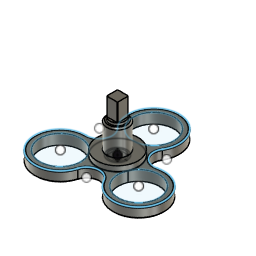
Base3 v0 (Autodesk Fusion 360 design; units mm, degrees)
Autodesk Fusion 360 part; units mm, degrees
sketch "Sketch1" plane through (0, 0, 0) normal (0, 0, 1) x (1, 0, 0)
  circle A0 centre (0, 0) radius 4
  circle A1 centre (0, 0) radius 1.5
  line L0 (0.98, 1.06) -> (-0.98, 1.06)
  line L1 (-1.06, 0.98) -> (-1.06, -0.98)
  line L2 (-0.98, -1.06) -> (0.98, -1.06)
  line L3 (1.06, -0.98) -> (1.06, 0.98)
  line L4 (1.06, 1.06) -> (-1.06, -1.06) construction
  line L5 (-1.06, 1.06) -> (1.06, -1.06) construction
  line L6 (0.98, 1.06) -> (1.06, 0.98)
  line L7 (-0.98, 1.06) -> (-1.06, 0.98)
  line L8 (-1.06, -0.98) -> (-0.98, -1.06)
  line L9 (1.06, -0.98) -> (0.98, -1.06)
  circle A2 centre (-0.8867, 7.9507) radius 4
  circle A3 centre (-6.4421, -4.7433) radius 4
  circle A4 centre (7.3289, -3.2074) radius 4
  arc A5 (-6.3446, 0.2558) -> (-4.4928, 4.4871) centre (-6.2958, 2.7553) ccw
  arc A6 (3.3938, 5.3667) -> (6.1323, 1.6473) centre (5.534, 4.0747) ccw
  arc A7 (2.9508, -5.6224) -> (-1.6396, -6.1344) centre (0.7617, -6.8299) ccw
  arc A8 (2.9508, -5.6224) -> (6.1323, 1.6473) centre (7.3289, -3.2074) ccw
  arc A9 (-6.3446, 0.2558) -> (-1.6396, -6.1344) centre (-6.4421, -4.7433) ccw
  arc A10 (3.3938, 5.3667) -> (-4.4928, 4.4871) centre (-0.8867, 7.9507) ccw
  circle A11 centre (0, 0) radius 1.8
  dimension "d1" = 8
  dimension "d2" = 3
  dimension "d3" = 2.12
  dimension "d4" = 2.12
  dimension "d5" = 0.08
  dimension "d6" = 0.08
  dimension "d7" = 0.08
  dimension "d8" = 0.08
  dimension "d9" = 0.08
  dimension "d10" = 0.08
  dimension "d11" = 0.08
  dimension "d12" = 0.08
  dimension "d13" = 8
  dimension "d18" = 360
  dimension "d19" = 10
  dimension "d20" = 5
  dimension "d23" = 5
  dimension "d24" = 5
  dimension "d31" = 3.6
  constraint coincident A0.centre A1.centre
  constraint concentric A0 A1
  constraint horizontal L0
  constraint perpendicular L0 L1
  constraint parallel L0 L2
  constraint parallel L1 L3
  constraint coincident L4 A0.centre
  constraint coincident L5 A0.centre
  constraint coincident L4.start L0
  constraint coincident L4.start L3
  constraint coincident L5.start L0
  constraint coincident L5.start L1
  constraint coincident L4.end L1
  constraint coincident L4.end L2
  constraint coincident L5.end L3
  constraint coincident L5.end L2
  constraint tangent A0 A2
  constraint concentric A2 A10
  constraint tangent A6 A10
  constraint tangent A6 A8
  constraint tangent A7 A8
  constraint tangent A7 A9
  constraint tangent A5 A10
  constraint tangent A5 A9
  constraint concentric A1 A11
  measures "d1" diameter of A0
  measures "d2" diameter of A1
  measures "d3" distance of L4.end L5.end
  measures "d4" distance of L5.start L4.end
  measures "d5" distance of L4.start L0.start
  measures "d6" distance of L4.start L3.end
  measures "d7" distance of L5.start L0.end
  measures "d8" distance of L5.start L1.start
  measures "d9" distance of L4.end L1.end
  measures "d10" distance of L4.end L2.start
  measures "d11" distance of L5.end L3.start
  measures "d12" distance of L5.end L2.end
  measures "d13" diameter of A2
  measures "d19" diameter of A10
  measures "d20" diameter of A6
  measures "d23" diameter of A7
  measures "d24" diameter of A5
  measures "d31" diameter of A11
extrude "Extrude1" add sketch "Sketch1" against normal blind 2 contours A5 A6 A7 A8 A9 A10 makes body 1
extrude "Extrude2" add sketch "Sketch1" along normal blind 10 separate body contours L0 L1 L2 L3 L6 L7 L8 L9 makes body 2
extrude "Extrude3" add sketch "Sketch1" along normal blind 6.5 contours A1 bodies 2
extrude "Extrude4" add sketch "Sketch1" along normal blind 6 contours A11 bodies 2
extrude "Extrude5" add sketch "Sketch1" along normal blind 1 contours A0 bodies 2 1
chamfer "Chamfer1" distance 0.2 distance2 0.2 6 edges at (11.9094, -5.212, 0) (3.5209, 2.5924, 0) (-1.4409, 12.9199, 0) (-4.0055, 1.753, 0) (-10.4685, -7.7078, 0) (0.4846, -4.3453, 0) measured on face at (-1.6264, -4.564, 0) measured on face at (3.144, 4.8081, -1.3333) measured on face at (-1.6264, -4.564, 0) measured on face at (-4.7482, 0.7919, -1.3333) measured on face at (-1.6264, -4.564, 0) measured on face at (-1.6025, -6.0174, -1.3333) on bodies 2
chamfer "Chamfer2" distance 0.2 angle 45 6 edges at (0.4846, -4.3453, -2) (-10.4685, -7.7078, -2) (-4.0055, 1.753, -2) (-1.4409, 12.9199, -2) (3.5209, 2.5924, -2) (11.9094, -5.212, -2) on bodies 2
move_face "OffsetFaces1" offset 0.3 1 faces at (1.7911, -0.1792, 4.3333) on bodies 2
chamfer "Chamfer3" distance 0.3 angle 45 1 edges at (-1.9579, -0.7594, 6) on bodies 2
equation "d6 = d5"
equation "d8 = d7"
equation "d10 = d9"
equation "d12 = d11"
